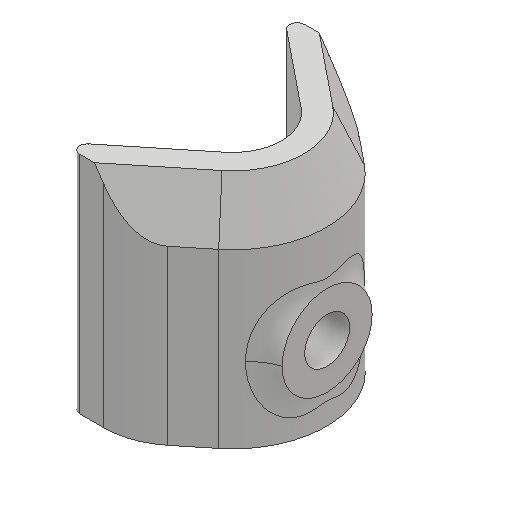
# Autodesk Inventor part: 3DP_ABS_Filament_Trash_Bin_Nozzle_Cleaner_Mount_MIR
Saved by Autodesk Inventor 2026.1 (Build 301233000, 233)
## iProperties
Created: 2016-12-23
Part Number: 3DP_ABS_Filament_Trash_Bin_Nozzle_Cleaner_Mount_MIR
Material: Ogólny
Document SubType Name: Modeling
Designer: Andrzej
Density: 1 g/cm^3
Appearance: Domyślna
Author: Andrzej
Autodesk Inventor part; units mm, degrees
ref_plane "XZ Plane" through (0, 0, 0) normal (0, 1, 0) x (-1, 0, 0)
ref_plane "XY Plane" through (0, 0, 0) normal (0, 0, 1) x (1, 0, 0)
sketch "Szkic1" plane through (0, 0, 0) normal (0, 0, 1) x (1, 0, 0)
  line L0 (-9.817, -10.5) -> (1.2567, -1.5559)
  arc A0 (1.2567, -1.5559) -> (1.2567, 1.5559) centre (0, 0) ccw
  line L1 (1.2567, 1.5559) -> (-9.817, 10.5)
  line L2 (-7.8276, -10.5) -> (2.0421, -2.5283)
  arc A1 (2.0421, -2.5283) -> (2.0421, 2.5283) centre (0, 0) ccw
  line L3 (2.0421, 2.5283) -> (-7.8276, 10.5)
  line L4 (-3.0531, -10.5) -> (3.9271, -4.8621)
  arc A2 (3.9271, -4.8621) -> (3.9271, 4.8621) centre (0, 0) ccw
  line L5 (3.9271, 4.8621) -> (-3.0531, 10.5)
  line L6 (-9.817, 10.5) -> (-3.0531, 10.5)
  line L7 (-9.817, -10.5) -> (-3.0531, -10.5)
  dimension "d0" = 1.25
  dimension "d1" = 3
  dimension "d9" = 3
  constraints: 16 end point, 6 point on circle, 3 centre point, 2 horizontal, 2 point on line
  measures "d0" distance between parallel lines of L0 L2
  measures "d1" distance between parallel lines of L2 L4
  measures "d9" distance between parallel lines of L5 L3
extrude "Wyciągnięcie proste1" add sketch "Szkic1" along normal blind 15 contours L2 A1 L3 L6 L5 A2 L4 L7
fillet "Zaokrąglenie1" radius 0.5 2 edges at (-7.8276, -10.5, 7.5) (-7.8276, 10.5, 7.5)
chamfer "Faza1" distance 1.5 distance2 3.5 3 edges at (0.437, -7.6811, 15) (6.25, 0, 15) (0.437, 7.6811, 15) measured on face at (0.1228, 7.2921, 15) measured on face at (0.1228, -7.2921, 15) measured on face at (5.75, 0, 15)
sketch "Szkic2" plane through (0, 0, 15) normal (0, 0, 1) x (1, 0, 0)
  line L0 (2.9846, -3.6952) -> (-5.4404, -10.5) projected
  arc A0 (2.9846, -3.6952) -> (2.9846, 3.6952) centre (0, 0) ccw projected
  line L1 (-5.4404, 10.5) -> (2.9846, 3.6952) projected
  line L2 (-5.4404, 10.5) -> (-6.4128, 10.5) projected
  arc A1 (-6.4128, 10.5) -> (-6.727, 9.611) centre (-6.4128, 10) ccw projected
  line L3 (-6.727, 9.611) -> (2.0421, 2.5283) projected
  arc A2 (2.0421, -2.5283) -> (2.0421, 2.5283) centre (0, 0) ccw projected
  line L4 (2.0421, -2.5283) -> (-6.727, -9.611) projected
  arc A3 (-6.727, -9.611) -> (-6.4128, -10.5) centre (-6.4128, -10) ccw projected
  line L5 (-6.4128, -10.5) -> (-5.4404, -10.5) projected
  line L6 (-3.0531, 10.5) -> (-5.4404, 10.5) projected
  line L7 (-5.4404, 10.5) -> (2.9846, 3.6952) projected
  line L8 (3.9271, 4.8621) -> (2.9846, 3.6952) projected
  line L9 (3.9271, 4.8621) -> (-3.0531, 10.5) projected
  line L10 (3.9271, 4.8621) -> (2.9846, 3.6952) projected
  arc A4 (2.9846, -3.6952) -> (2.9846, 3.6952) centre (0, 0) ccw projected
  line L11 (3.9271, -4.8621) -> (2.9846, -3.6952) projected
  arc A5 (3.9271, -4.8621) -> (3.9271, 4.8621) centre (0, 0) ccw projected
  line L12 (-5.4404, -10.5) -> (-3.0531, -10.5) projected
  line L13 (-3.0531, -10.5) -> (3.9271, -4.8621) projected
  line L14 (3.9271, -4.8621) -> (2.9846, -3.6952) projected
  line L15 (2.9846, -3.6952) -> (-5.4404, -10.5) projected
  line L16 (-14.2058, 7.5) -> (11.6148, 7.5)
  line L17 (-12.3296, -7.5) -> (12.9848, -7.5)
  line L18 (-14.2058, 7.5) -> (-14.2058, 15.6516)
  line L19 (-14.2058, 15.6516) -> (11.3655, 15.6516)
  line L20 (11.3655, 15.6516) -> (11.6148, 7.5)
  line L21 (12.9848, -7.5) -> (13.6668, -18.6215)
  line L22 (13.6668, -18.6215) -> (-13.9485, -13.7372)
  line L23 (-13.9485, -13.7372) -> (-12.3296, -7.6811)
  line L24 (-12.3296, -7.6811) -> (-12.3296, -7.5)
  dimension "d13" = 7.5
  dimension "d14" = 7.5
  constraints: 18 end point, 2 horizontal, 2 perpendicular, 1 vertical
  measures "d13" distance from line of L16 point (0, 0)
  measures "d14" distance from line of L17 point (0, 0)
extrude "Wyciągnięcie proste2" cut sketch "Szkic2" against normal through all contours L17 L13 L12 L0 | L0 L5 A3 L4 L17 | L12 L13 L17 L21 L22 L23 L24 L4 A3 L5 | L16 L3 A1 L2 L1 | L1 L6 L9 L16 | L2 A1 L3 L16 L18 L19 L20 L9 L6
fillet "Zaokrąglenie3" radius 5 2 edges at (0.6612, -7.5, 5.75) (0.6612, 7.5, 5.75)
ref_plane "Płaszczyzna konstrukcyjna1" through (6.3, 0, 0) normal (1, 0, 0) x (0, 1, 0)
sketch "Szkic3" plane through (6.3, 0, 0) normal (1, 0, 0) x (0, 1, 0)
  ellipse E0 centre (2.5, 23.1667) end of major axis (6.644, 11.5427) minor radius 2.9701 (6.3897, 11.5) -> (7.5, 14.0907) ccw projected
  line L0 (6.3897, 11.5) -> (6.3897, 0) projected
  line L1 (6.3897, 0) -> (7.5, 0) projected
  line L2 (7.5, 0) -> (7.5, 14.0907) projected
  line L3 (6.3897, 11.5) -> (6.3897, 0) projected
  line L4 (4.8621, 11.5) -> (6.3897, 11.5) projected
  line L5 (4.8621, 0) -> (4.8621, 11.5) projected
  line L6 (4.8621, 0) -> (6.3897, 0) projected
  line L7 (-4.8621, 11.5) -> (4.8621, 11.5) projected
  line L8 (-4.8621, 0) -> (-4.8621, 11.5) projected
  line L9 (-4.8621, 0) -> (4.8621, 0) projected
  line L10 (4.8621, 0) -> (4.8621, 11.5) projected
  line L11 (-6.3897, 0) -> (-6.3897, 11.5) projected
  line L12 (-6.3897, 0) -> (-4.8621, 0) projected
  line L13 (-4.8621, 0) -> (-4.8621, 11.5) projected
  line L14 (-6.3897, 11.5) -> (-4.8621, 11.5) projected
  line L15 (-7.5, 0) -> (-6.3897, 0) projected
  line L16 (-6.3897, 0) -> (-6.3897, 11.5) projected
  ellipse E1 centre (-2.5, 23.1667) end of major axis (-6.644, 11.5427) minor radius 2.9701 (-7.5, 14.0907) -> (-6.3897, 11.5) ccw projected
  line L17 (-7.5, 14.0907) -> (-7.5, 0) projected
  line L18 (4.8621, 11.5) -> (3.6952, 15) projected
  line L19 (3.6952, 15) -> (-3.6952, 15) projected
  line L20 (-4.8621, 11.5) -> (-3.6952, 15) projected
  line L21 (-4.8621, 11.5) -> (4.8621, 11.5) projected
  ellipse E2 centre (-2.5, 23.1667) end of major axis (-6.644, 11.5427) minor radius 2.9701 (-7.5, 14.0907) -> (-6.3897, 11.5) ccw projected
  line L22 (-6.3897, 11.5) -> (-4.8621, 11.5) projected
  line L23 (-4.8621, 11.5) -> (-3.6952, 15) projected
  line L24 (-3.6952, 15) -> (-7.5, 15) projected
  line L25 (-7.5, 15) -> (-7.5, 14.0907) projected
  ellipse E3 centre (2.5, 23.1667) end of major axis (6.644, 11.5427) minor radius 2.9701 (6.3897, 11.5) -> (7.5, 14.0907) ccw projected
  line L26 (7.5, 14.0907) -> (7.5, 15) projected
  line L27 (7.5, 15) -> (3.6952, 15) projected
  line L28 (4.8621, 11.5) -> (3.6952, 15) projected
  line L29 (4.8621, 11.5) -> (6.3897, 11.5) projected
  circle A0 centre (0, 5) radius 3
  point P0 (0, 0)
  dimension "d19" = 10
  dimension "d20" = 7.5
  dimension "d21" = 7.5
  dimension "d22" = 6
  constraints: 1 centre point, 1 coincident, 4 other
  measures "d19" distance from line of L19 point (0, 5)
  measures "d20" distance from line of L17 point (0, 5)
  measures "d21" distance from line of L2 point (0, 5)
  measures "d22" diameter of A0
extrude "Wyciągnięcie proste3" add sketch "Szkic3" against normal blind 1 contours A0
hole "Otwór1" at (6.3, 0, 5) direction (-1, 0, 0) diameter 3 depth 8 tip angle 118
fillet "Zaokrąglenie4" radius 3 1 edges at (5.4829, -3, 5.0007)
fillet "Zaokrąglenie5" radius 0.5 2 edges at (-4.1133, -7.5, 7.5) (-4.1133, 7.5, 7.5)
equation "\"d9\" = d1"
equation "\"d14\" = d13"
